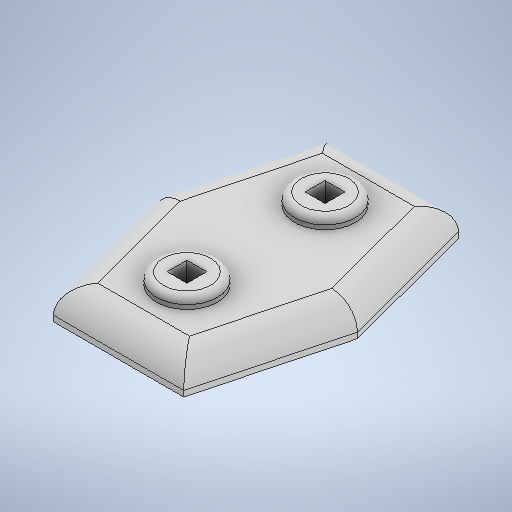
# Autodesk Inventor part: Part2
Saved by Autodesk Inventor 2025.3 (Build 293356000, 356)
## iProperties
Created: 2025-07-14
Part Number: Part2
Material: Generic
Document SubType Name: Modeling
Designer: steve
Density: 1 g/cm^3
Appearance: Default
Author: steve
Autodesk Inventor part; units mm, degrees
ref_plane "YZ Plane" through (0, 0, 0) normal (1, 0, 0) x (0, 1, 0)
ref_plane "XZ Plane" through (0, 0, 0) normal (0, 1, 0) x (-1, 0, 0)
ref_plane "XY Plane" through (0, 0, 0) normal (0, 0, 1) x (1, 0, 0)
sketch "Sketch1" plane through (0, 0, 0) normal (0, 1, 0) x (-1, 0, 0)
  line L0 (0, 9.9) -> (0, -9.9)
  line L1 (-4.7, 9.9) -> (4.7, 9.9)
  line L2 (0, 0) -> (7.31, 0)
  line L3 (4.7, 9.9) -> (7.31, 0)
  line L4 (0, 0) -> (-7.31, 0)
  line L5 (-4.7, 9.9) -> (-7.31, 0)
  line L6 (-4.7, -9.9) -> (4.7, -9.9)
  line L7 (4.7, -9.9) -> (7.31, 0)
  line L8 (-4.7, -9.9) -> (-7.31, 0)
  line L9 (0, 9.9) -> (0, 5.69)
  line L10 (0, 5.69) -> (0.715, 5.69)
  line L11 (0.715, 5.69) -> (0.715, 4.26)
  line L12 (0.715, 4.26) -> (-0.715, 4.26)
  line L13 (-0.715, 4.26) -> (-0.715, 5.69)
  line L14 (-0.715, 5.69) -> (0, 5.69)
  circle A0 centre (0, 4.975) radius 2.2
  line L15 (0, -5.69) -> (0.715, -5.69)
  line L16 (0.715, -5.69) -> (0.715, -4.26)
  line L17 (0.715, -4.26) -> (-0.715, -4.26)
  line L18 (-0.715, -4.26) -> (-0.715, -5.69)
  line L19 (-0.715, -5.69) -> (0, -5.69)
  circle A1 centre (0, -4.975) radius 2.2
  point P0 (0, -9.9)
  dimension "d0" = 19.8
  dimension "d1" = 0
  dimension "d2" = 0
  dimension "d3" = 9.4
  dimension "d5" = 7.31
  dimension "d6" = 4.21
  dimension "d7" = 0.715
  dimension "d8" = 1.43
  dimension "d9" = 1.43
  dimension "d10" = 4.4
  constraints: 40 end point, 11 symmetric about line, 5 perpendicular, 4 midpoint, 4 point on line, 2 centre point, 2 horizontal, 1 vertical, 1 other
  measures "d0" distance of L0.start L0.end
  measures "d1" distance of point (0, 0) L2.start
  measures "d2" distance from line of point (0, 0) L0
  measures "d3" distance of L1.start L1.end
  measures "d5" distance of L2.start L2.end
  measures "d6" distance of L9.start L9.end
  measures "d7" distance of L9.end L10.end
  measures "d8" distance of L10.end L11.end
  measures "d9" distance of L11.end L12.end
  measures "d10" diameter of A0
extrude "Extrusion1" add sketch "Sketch1" against normal blind 2.21 contours L1 L3 L2 L0 A0 | L0 A0 L4 L5 L1 | L4 L0 A1 L6 L8 | L7 L6 L0 A1 L2
extrude "Extrusion2" add sketch "Sketch1" against normal blind 2.21 contours A0 L0 L12 L11 L10 | L0 L14 L13 L12 A0 | A1 L0 L15 L16 L17 | L0 L17 L18 L19 A1
extrude "Extrusion3" add sketch "Sketch1" along normal blind 0.8 contours A0 L0 L12 L11 L10 | L0 L14 L13 L12 A0 | A1 L0 L15 L16 L17 | L0 L17 L18 L19 A1
fillet "Fillet1" radius 0.5 1 edges at (2.2, 0.8, 4.975)
fillet "Fillet2" radius 0.5 1 edges at (2.2, 0.8, -4.975)
fillet "Fillet3" radius 1.8 6 edges at (6.005, 0, -4.95) (6.005, 0, 4.95) (0, 0, -9.9) (-6.005, 0, -4.95) (-6.005, 0, 4.95) (0, 0, 9.9)
body "Solid1"
